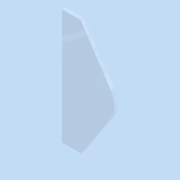
# Autodesk Inventor part: 본체 창
Saved by Autodesk Inventor 2020 (Build 240168000, 168)
## iProperties
Created: 2020-05-05
Part Number: 본체 창
Material: 일반
Document SubType Name: Modeling
Designer: sbahn
Density: 1 g/cm^3
Appearance: 선명
Author: sbahn
Autodesk Inventor part; units mm, degrees
ref_plane "YZ Plane" through (0, 0, 0) normal (1, 0, 0) x (0, 1, 0)
ref_plane "XZ Plane" through (0, 0, 0) normal (0, 1, 0) x (-1, 0, 0)
ref_plane "XY Plane" through (0, 0, 0) normal (0, 0, 1) x (1, 0, 0)
sketch "스케치1" plane through (0, 0, 0) normal (0, 0, 1) x (1, 0, 0)
  line L0 (-11.461, -6.8509) -> (-28.6226, -32.9687) projected
  line L1 (-28.6226, -32.9687) -> (-39.2674, -32.97) projected
  line L2 (-39.2674, -32.97) -> (-39.2674, 33) projected
  spline S0 degree 3 poles (-11.4533, 6.8391) (-11.0054, 6.1558) (-10.3404, 4.893) (-9.8386, 3.359) (-9.5769, 2.184) (-9.4603, 1.3908) (-9.3876, 0.3933) (-9.388, -0.4071) (-9.4619, -1.4045) (-9.5794, -2.1975) (-9.7985, -3.1765) (-10.0312, -3.9474) (-10.392, -4.8896) (-10.8218, -5.8074) (-11.2367, -6.5094) (-11.461, -6.8509) knots -3.699059 -3.699059 -3.699059 -3.699059 -3.513059 -3.373559 -3.327059 -3.234059 -3.187559 -3.094559 -3.048059 -2.955059 -2.908559 -2.815559 -2.769059 -2.676059 -2.583059 -2.583059 -2.583059 -2.583059 projected
  line L3 (-28.6226, -32.9687) -> (-28.6226, 33)
  line L4 (-28.6226, 33) -> (-39.2674, 33)
  line L5 (-28.6226, 33) -> (-11.4533, 6.8391)
  point P0 (0, 0)
  constraints: 6 end point, 1 perpendicular, 1 vertical
extrude "돌출1" add sketch "스케치1" against normal blind 2
